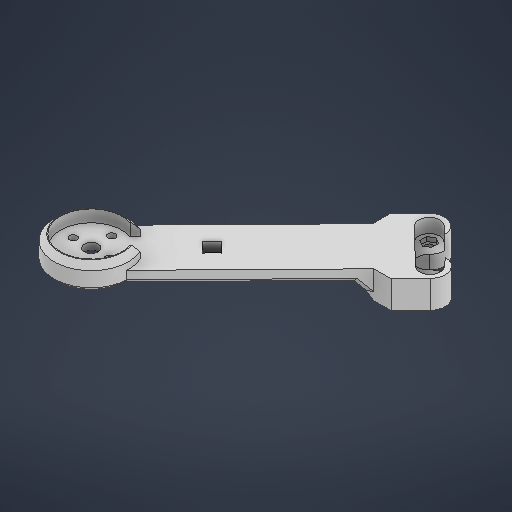
# Autodesk Inventor part: Drone_arm
Saved by Autodesk Inventor 2026.1 (Build 301233000, 233)
## iProperties
Created: 2025-07-26
Part Number: Drone_arm
Material: Generic
Document SubType Name: Modeling
Designer: rohit
Density: 1 g/cm^3
Appearance: Default
Author: rohit
Autodesk Inventor part; units mm, degrees
ref_plane "YZ Plane" through (0, 0, 0) normal (1, 0, 0) x (0, 1, 0)
ref_plane "Work Plane2" through (0, 1.599999, 0) normal (0, 1, 0) x (1, 0, 0)
sketch "Sketch2" plane through (0, 1.599999, 0) normal (0, 1, 0) x (1, 0, 0)
  line L0 (0, 0) -> (120.000013, 0.000002)
  line L1 (-0.000001, 100.000056) -> (0, 0)
  circle A0 centre (23.000003, 7.000013) radius 1.749996
  arc A1 (11.825466, 17.944839) -> (18.000765, 11.896484) centre (14.466612, 14.464787) ccw
  line L2 (23.000003, 7.000013) -> (27.999242, 2.103543)
  line L3 (6.445161, 23.214543) -> (1.808844, 27.755553)
  arc A2 (11.825466, 17.944839) -> (1.808844, 27.755553) centre (6.817155, 22.850196) ccw
  arc A3 (27.999242, 2.103544) -> (18.000765, 11.896484) centre (23.000003, 7.000014) ccw
  line L4 (27.999242, 2.103544) -> (23.000003, 7.000014)
  line L5 (27.999242, 2.103544) -> (19.112725, -6.969484)
  line L6 (1.808844, 27.755553) -> (-7.077672, 18.682525)
  line L7 (23.000003, 7.000014) -> (6.817155, 22.850196)
  line L8 (23.000003, 7.000014) -> (14.908876, 14.924814)
  line L9 (14.908876, 14.924814) -> (-73.956283, -75.805464)
  line L10 (27.999242, 2.103544) -> (1.808844, 27.755553)
  line L11 (-73.956283, -75.805464) -> (22.671338, 22.850196)
  line L12 (-62.015027, -63.613583) -> (-68.56021, -57.202948)
  circle A4 centre (-62.015027, -63.613583) radius 17.065625
  circle A5 centre (-62.015027, -63.613583) radius 13.890625
  line L13 (-59.1468, -42.535186) -> (-63.111626, -46.583227)
  line L14 (-59.1468, -42.535186) -> (-6.994891, 10.711297)
  line L15 (-7.077672, 18.682525) -> (-6.994891, 10.711297)
  line L16 (-41.000744, -60.308218) -> (-44.96557, -64.356259)
  line L17 (19.112725, -6.969484) -> (11.160634, -7.052067)
  line L18 (-41.000744, -60.308218) -> (11.160634, -7.052067)
  circle A6 centre (6.817155, 22.850196) radius 1.749996
  dimension "d26" = 4.3688
  dimension "d28" = 12.7
  dimension "d29" = 12.7
  dimension "d30" = 90
  dimension "d31" = 90
  dimension "d32" = 15.85018
  dimension "d33" = 7.9248
  dimension "d35" = 6.9977
  dimension "d36" = 7.0104
  dimension "d37" = 127
  dimension "d38" = 90
  dimension "d40" = 17.06563
  dimension "d41" = 27.78125
  dimension "d205" = 3.49999
  constraints: 34 end point, 9 point on circle, 6 centre point, 4 coincident, 2 point on line, 2 tangent, 1 perpendicular
  measures "d26" radius of A1
  measures "d28" distance of L4.start L5.end
  measures "d29" distance of L3.end L6.end
  measures "d30" angle of L3 L6
  measures "d31" angle of L5 L2
  measures "d32" vertical distance of L4.end L7.end
  measures "d33" vertical distance of L4.end L8.end
  measures "d35" radius of A3
  measures "d36" radius of A2
  measures "d37" distance of L8.end L9.end
  measures "d38" angle of L7 L9
  measures "d40" distance from line of L12 L9.end
  measures "d41" diameter of A5
  measures "d205" diameter of A6
extrude "Extrusion2" add sketch "Sketch2" along normal blind 12.7 contours L1 L6 L3 A6 L7 A1 L9 L0 | L0 L9 A4 L13 L14 L15 L6 L1 | L9 A1 L7 A0 L2 L5 L0 | L0 L5 L17 L18 L16 A4 L9 | A4 L9 A5 | L9 A5 A4 | A2 L7 A6 L3 | L2 A0 L7 A3 | A5 L9 | L9 A5
ref_plane "Work Plane3" through (0, 14.299999, 0) normal (0, 1, 0) x (1, 0, 0)
sketch "Sketch6" plane through (0, 14.299999, 0) normal (0, 1, 0) x (1, 0, 0)
  circle A0 centre (6.817155, 22.850196) radius 1.749996
  line L0 (6.817155, 24.600192) -> (6.817155, 22.850196)
  circle A1 centre (23.000003, 7.000013) radius 1.749996
  line L1 (23.000003, 8.75001) -> (23.000003, 7.000013)
  circle A2 centre (6.817155, 22.850196) radius 1.749996
  circle A3 centre (23.000003, 7.000013) radius 1.749997
  circle A4 centre (6.817155, 22.850196) radius 4.7879
  circle A5 centre (23.000003, 7.000013) radius 4.7879
  line L2 (6.817155, 22.850196) -> (10.237979, 26.200114)
  line L3 (6.817155, 22.850196) -> (32.808158, 22.850196)
  line L4 (23.000003, 7.000013) -> (26.38556, 10.38557)
  line L5 (26.38556, 10.38557) -> (10.237979, 26.200114)
  line L6 (10.095065, 26.34008) -> (3.466978, 19.429626)
  line L7 (26.38556, 10.38557) -> (19.614447, 3.614457)
  line L8 (19.614447, 3.614457) -> (3.466978, 19.429626)
  arc A6 (11.825466, 17.944839) -> (1.808844, 27.755553) centre (6.817155, 22.850196) ccw
  line L9 (10.095065, 26.34008) -> (13.827555, 22.850196)
  arc A7 (27.999242, 2.103544) -> (18.000765, 11.896484) centre (23.000003, 7.000014) ccw
  line L10 (23.000003, 7.000014) -> (23.000003, 28.445518)
  line L11 (26.38556, 10.38557) -> (23.000003, 13.997714)
  point P0 (0, 0)
  point P1 (26.314279, 10.45538)
  point P2 (22.703753, 13.991441)
  point P3 (13.825642, 22.686445)
  dimension "d61" = 9.5758
  dimension "d62" = 9.5758
  dimension "d63" = 44.4
  dimension "d64" = 45
  constraints: 24 end point, 7 point on circle, 4 coincident, 4 point on line, 4 vertical alignment, 2 centre point, 2 vertical, 1 horizontal, 1 perpendicular, 1 tangent, 6 other
  measures "d61" diameter of A4
  measures "d62" diameter of A5
  measures "d63" angle of L2 L3
  measures "d64" angle of L1 L4
sketch "Sketch7" plane through (0, 14.299999, 0) normal (0, 1, 0) x (1, 0, 0)
  arc A0 (-63.111626, -46.583227) -> (-44.96557, -64.356259) centre (-62.015027, -63.613583) ccw
  circle A1 centre (-62.015027, -63.613583) radius 17.065625
  circle A2 centre (-62.015027, -63.613583) radius 14.144625
  point P0 (0, 0)
  point P1 (-44.96557, -64.356259)
  dimension "d67" = 28.28925
  constraints: 2 centre point, 2 coincident
  measures "d67" diameter of A2
extrude "Extrusion5" add sketch "Sketch7" along normal blind 5.55625
chamfer "Chamfer4" distance 2.54 angle 45 1 edges at (-79.0645, 19.8562, 62.8709)
extrude "Extrusion7" cut sketch "Sketch6" against normal blind 6.4262 contours L3 A4 L6 A0 | A0 L2 A4 L3 | A0 L6 A4 L2 | L6 A4 A0 | L3 L5 L10 A5 L8 A4 | A4 L5 L3 | A4 L9 L3 L5 | L3 A6 L5 | L7 A1 L4 A5 | A5 L10 A1 L7 | L5 L10 L11 | L10 L5 A5 | A5 L4 A1 L10 | A7 L10 L5
sketch "Sketch9" plane through (0, 14.299999, 0) normal (0, 1, 0) x (1, 0, 0)
  line L0 (0, 0) -> (0, 56.563662)
  arc A0 (-61.745166, -49.72558) -> (-48.135624, -63.055354) centre (-62.015027, -63.613583) ccw
  line L1 (-62.015027, -63.613583) -> (-50.053464, -51.437174)
  line L2 (-50.053464, -51.437174) -> (-36.703505, -37.847432)
  line L3 (-36.703505, -37.847432) -> (-34.438548, -40.072425)
  line L4 (-36.703505, -37.847432) -> (-38.968462, -35.622438)
  line L5 (-38.968462, -35.622438) -> (-34.517758, -31.093229)
  line L6 (-34.517758, -31.093229) -> (-30.067772, -35.623143)
  line L7 (-30.067772, -35.623143) -> (-34.438548, -40.072425)
  line L8 (-62.015027, -63.613583) -> (-36.703505, -37.847432)
  line L9 (-32.293118, -33.357828) -> (26.984699, 26.984699)
  dimension "d86" = 127
  dimension "d87" = 17.0688
  dimension "d88" = 19.05
  constraints: 20 end point, 3 perpendicular, 3 point on line, 1 vertical
  measures "d86" distance of L1.start L9.end
  measures "d87" distance of L1.start L1.end
  measures "d88" distance of L1.end L2.end
extrude "Extrusion8" cut sketch "Sketch9" against normal blind 25.4
sketch "Sketch10" plane through (0, 14.299999, 0) normal (0, 1, 0) x (1, 0, 0)
  arc A0 (-44.96557, -64.356259) -> (-63.111626, -46.583227) centre (-62.015027, -63.613583) ccw
  line L0 (-62.015027, -63.613583) -> (-62.015027, 15.913848)
  arc A1 (-63.111626, -46.583227) -> (-44.96557, -64.356259) centre (-62.015027, -63.613583) ccw
  line L1 (-62.015027, -63.613583) -> (49.774543, 48.175988)
  line L2 (-62.015027, -63.613583) -> (-49.945563, -51.544119)
  line L3 (-49.945563, -51.544119) -> (-52.014859, -53.613414)
  line L4 (-49.945563, -51.544119) -> (-47.700499, -53.789183)
  line L5 (-52.190627, -49.299055) -> (-47.700499, -53.789183)
  line L6 (-56.231743, -53.34017) -> (-51.741614, -57.830298)
  line L7 (-53.986679, -55.585234) -> (-49.49655, -60.075362)
  line L8 (-53.986679, -55.585234) -> (-58.476807, -51.095106)
  line L9 (-49.49655, -60.075362) -> (-45.455435, -56.034247)
  line L10 (-58.476807, -51.095106) -> (-54.435691, -47.053991)
  line L11 (-54.435691, -47.053991) -> (-45.455435, -56.034247)
  point P0 (0, 0)
  dimension "d95" = 45
  dimension "d96" = 17.0688
  dimension "d112" = 5.715
  constraints: 24 end point, 4 point on line, 2 perpendicular, 1 collinear, 1 midpoint, 1 vertical
  measures "d95" angle of L1 L0
  measures "d96" distance of L1.start L2.end
  measures "d112" distance of L8.end L10.end
sketch "Sketch12" plane through (0, 14.299999, 0) normal (0, 1, 0) x (1, 0, 0)
  arc A0 (-61.745166, -49.72558) -> (-48.135624, -63.055354) centre (-62.015027, -63.613583) ccw
  line L0 (-62.015027, -63.613583) -> (-62.015027, -25.183196)
  circle A1 centre (-62.015027, -63.613583) radius 3.175
  point P0 (0, 0)
  dimension "d106" = 6.35
  constraints: 2 end point, 1 centre point, 1 coincident, 1 vertical
  measures "d106" diameter of A1
extrude "Extrusion10" cut sketch "Sketch12" against normal blind 25.4
extrude "Extrusion11" cut sketch "Sketch10" along normal blind 25.4 contours L9 L7 L6 L1 A0 | A0 L4 L11 L9 | L1 L6 L8 L10 A0 | A0 L10 L11 L5
sketch "Sketch15" plane through (11.160634, 1.599999, 7.052067) normal (0.7144116, 0, 0.6997257) x (0.6997257, 0, -0.7144116)
  line L0 (5.623281, 0) -> (-0.013532, 0)
  line L1 (-0.013532, 0) -> (-23.040543, 23.027011)
  line L2 (-80.211727, 0) -> (0, 0)
  line L3 (-0.013532, 0) -> (-0.013532, 12.7)
  line L4 (-0.013532, 0) -> (-6.363532, 0)
  line L5 (-108.676719, 0) -> (-108.676719, 15.71625)
  line L6 (-108.676719, 6.35) -> (-6.363532, 6.35)
  line L7 (-108.676719, 6.35) -> (-108.676719, 0)
  line L8 (-108.676719, 0) -> (-0.013532, 0)
  point P0 (-2.771303, -1.599999)
  point P1 (-80.211727, 0)
  dimension "d125" = 45
  dimension "d126" = 6.35
  constraints: 10 end point, 5 point on line, 1 collinear, 1 perpendicular
  measures "d125" angle of L2 L1
  measures "d126" distance of L0.end L4.end
extrude "Extrusion13" cut sketch "Sketch15" along normal mid plane 76.2
sketch "Sketch16" plane through (6.707907, 7.949999, 11.598248) normal (0, -1, 0) x (0.7144116, 0, 0.6997257)
  circle A0 centre (-12.7, 85.247562) radius 3.175
  line L0 (-12.7, 85.247562) -> (-5.982481, 91.965081)
  line L1 (-12.7, 85.247562) -> (-6.901718, 79.44928)
  line L2 (-12.7, 85.247562) -> (-18.498282, 91.045844)
  line L3 (-12.7, 85.247562) -> (-19.417519, 78.530043)
  circle A1 centre (-5.982481, 91.965081) radius 1.749996
  circle A2 centre (-6.901718, 79.44928) radius 1.749997
  circle A3 centre (-19.417519, 78.530043) radius 1.749996
  circle A4 centre (-18.498282, 91.045844) radius 1.749997
  point P0 (-12.907799, -3.592229)
  dimension "d187" = 9.50001
  dimension "d188" = 8.20001
  dimension "d189" = 8.20001
  dimension "d190" = 9.50001
  dimension "d191" = 90
  dimension "d192" = 90
  dimension "d193" = 90
  dimension "d195" = 3.49999
  dimension "d196" = 3.49999
  dimension "d197" = 3.49999
  dimension "d198" = 3.49999
  constraints: 8 end point, 4 centre point, 4 coincident
  measures "d187" distance of L0.start L0.end
  measures "d188" distance of L0.start L1.end
  measures "d189" distance of L0.start L2.end
  measures "d190" distance of L0.start L3.end
  measures "d191" angle of L1 L0
  measures "d192" angle of L0 L2
  measures "d193" angle of L2 L3
  measures "d195" diameter of A1
  measures "d196" diameter of A2
  measures "d197" diameter of A3
  measures "d198" diameter of A4
sketch "Sketch17" plane through (6.707907, 7.949999, 11.598248) normal (0, -1, 0) x (0.7144116, 0, 0.6997257)
  circle A0 centre (-12.7, 85.247562) radius 3.175
  circle A1 centre (-12.7, 85.247562) radius 14.144625
  point P0 (-12.907799, -3.592229)
  dimension "d137" = 28.28925
  constraints: 1 centre point, 1 coincident
  measures "d137" diameter of A1
extrude "Extrusion14" cut sketch "Sketch17" against normal blind 3.175
chamfer "Chamfer5" distance 2.54 angle 45 5 edges at (-73.9563, 7.95, 75.8055) (-19.1288, 7.95, 37.9773) (-37.2749, 7.95, 20.2042) (-9.2165, 4.775, -8.443) (8.9295, 4.775, 9.33)
sketch "Sketch18" plane through (0, 7.873799, 0) normal (0, 1, 0) x (1, 0, 0)
  circle A0 centre (23.000003, 7.000013) radius 1.749996
  line L0 (23.000003, 7.000013) -> (23.000003, 3.825013)
  line L1 (23.000003, 7.000013) -> (20.250373, 5.412513)
  line L2 (23.000003, 7.000013) -> (20.250373, 8.587513)
  line L3 (23.000003, 7.000013) -> (23.000003, 10.175013)
  line L4 (23.000003, 7.000013) -> (25.749634, 8.587513)
  line L5 (23.000003, 7.000013) -> (25.749634, 5.412513)
  line L6 (23.000003, 3.825013) -> (25.749634, 5.412513)
  line L7 (25.749634, 8.587513) -> (25.749634, 5.412513)
  line L8 (25.749634, 8.587513) -> (23.000003, 10.175013)
  line L9 (23.000003, 10.175013) -> (20.250373, 8.587513)
  line L10 (20.250373, 8.587513) -> (20.250373, 5.412513)
  line L11 (20.250373, 5.412513) -> (23.000003, 3.825013)
  circle A1 centre (6.817155, 22.850196) radius 1.749996
  line L12 (6.817155, 22.850196) -> (6.817155, 26.025196)
  line L13 (6.817155, 22.850196) -> (9.566786, 24.437696)
  line L14 (6.817155, 22.850196) -> (9.566786, 21.262696)
  line L15 (6.817155, 22.850196) -> (6.817155, 19.675196)
  line L16 (6.817155, 22.850196) -> (4.067524, 21.262696)
  line L17 (6.817155, 22.850196) -> (4.067524, 24.437696)
  line L18 (6.817155, 19.675196) -> (4.067524, 21.262696)
  line L19 (4.067524, 21.262696) -> (4.067524, 24.437696)
  line L20 (6.817155, 26.025196) -> (4.067524, 24.437696)
  line L21 (9.566786, 24.437696) -> (6.817155, 26.025196)
  line L22 (9.566786, 24.437696) -> (9.566786, 21.262696)
  line L23 (6.817155, 19.675196) -> (9.566786, 21.262696)
  point P0 (0, 0)
  dimension "d158" = 3.175
  dimension "d163" = 3.175
  dimension "d165" = 60
  dimension "d167" = 3.175
  dimension "d168" = 3.175
  dimension "d169" = 3.175
  dimension "d170" = 3.175
  dimension "d171" = 60
  dimension "d172" = 60
  dimension "d173" = 60
  dimension "d174" = 60
  dimension "d175" = 3.175
  dimension "d176" = 3.175
  dimension "d177" = 3.175
  dimension "d178" = 3.175
  dimension "d179" = 3.175
  dimension "d180" = 3.175
  dimension "d181" = 60
  dimension "d182" = 60
  dimension "d183" = 60
  dimension "d184" = 60
  constraints: 48 end point, 2 parallel, 2 vertical, 1 point on line
  measures "d158" distance of L0.start L1.end
  measures "d163" distance of L0.start L0.end
  measures "d165" angle of L0 L1
  measures "d167" distance of L0.start L2.end
  measures "d168" distance of L0.start L3.end
  measures "d169" distance of L0.start L4.end
  measures "d170" distance of L0.start L5.end
  measures "d171" angle of L2 L1
  measures "d172" angle of L5 L0
  measures "d173" angle of L4 L5
  measures "d174" angle of L3 L4
  measures "d175" distance of L12.start L12.end
  measures "d176" distance of L12.start L13.end
  measures "d177" distance of L12.start L14.end
  measures "d178" distance of L12.start L15.end
  measures "d179" distance of L12.start L16.end
  measures "d180" distance of L12.start L17.end
  measures "d181" angle of L17 L16
  measures "d182" angle of L12 L17
  measures "d183" angle of L13 L12
  measures "d184" angle of L14 L13
extrude "Extrusion16" cut sketch "Sketch18" against normal blind 2.000001 contours A0 L4 L7 L5 | A0 L3 L8 L4 | L5 L6 L0 A0 | A0 L2 L9 L3 | L0 L11 L1 A0 | A0 L1 L10 L2 | A1 L13 L22 L14 | A1 L12 L21 L13 | L14 L23 L15 A1 | A1 L17 L20 L12 | L15 L18 L16 A1 | A1 L16 L19 L17
extrude "Extrusion17" cut sketch "Sketch16" against normal blind 8.200009 contours A1 | A2 | A3 | A4
body "Solid1"
